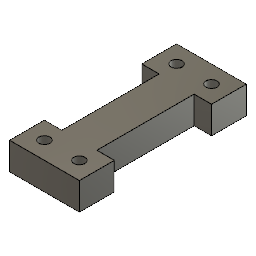
spacer_for_lbt-131_2mm (Autodesk Fusion 360 design; units mm, degrees)
Autodesk Fusion 360 part; units mm, degrees
note: some values were not read from the file. Set by a fixed rule: which sketch regions a step uses.
sketch "スケッチ1" plane through (0, 0, 0) normal (0, 1, 0) x (1, 0, 0)
  line L0 (0, 0) -> (0, 4.8)
  line L1 (0, 4.8) -> (1.27, 4.8)
  circle A0 centre (1.27, 4.8) radius 0.4
  circle A1 centre (-1.27, 4.8) radius 0.4
  circle A2 centre (-1.27, -4.8) radius 0.4
  circle A3 centre (1.27, -4.8) radius 0.4
  line L2 (-2.54, 3.53) -> (0, 3.53)
  line L3 (0, 3.53) -> (0, 6.07)
  line L4 (0, 6.07) -> (-2.54, 6.07)
  line L5 (-2.54, 6.07) -> (-2.54, 3.53)
  line L6 (-2.54, 3.53) -> (0, 6.07) construction
  line L7 (0, 3.53) -> (-2.54, 6.07) construction
  line L8 (2.54, 3.53) -> (0, 3.53)
  line L9 (2.54, 6.07) -> (2.54, 3.53)
  line L10 (0, 6.07) -> (2.54, 6.07)
  line L11 (0, 0) -> (1.27, 0)
  line L12 (-2.54, -3.53) -> (0, -3.53)
  line L13 (-2.54, -6.07) -> (-2.54, -3.53)
  line L14 (0, -6.07) -> (-2.54, -6.07)
  line L15 (0, -6.07) -> (2.54, -6.07)
  line L16 (2.54, -6.07) -> (2.54, -3.53)
  line L17 (2.54, -3.53) -> (0, -3.53)
  line L18 (1.27, 0) -> (1.27, 3.53)
  line L19 (-1.27, 0) -> (-1.27, 3.53)
  line L20 (1.27, 0) -> (1.27, -3.53)
  line L21 (-1.27, 0) -> (-1.27, -3.53)
  point P0 (-1.27, 4.8)
  dimension "d1" = 4.8
  dimension "d2" = 1.27
  dimension "d3" = 0.8
  dimension "d4" = 2.54
  dimension "d5" = 2.54
  dimension "d6" = 1.27
  constraint coincident L0.start L11.start
  constraint vertical L0
  constraint perpendicular L0 L1
  constraint coincident L1.end A0.centre
  constraint symmetric L0 A0 A1
  constraint perpendicular L2 L3
  constraint parallel L2 L4
  constraint parallel L3 L5
  constraint horizontal L2
  constraint coincident L6 P0
  constraint coincident L7 P0
  constraint coincident P0 A1.centre
  constraint symmetric L0 L2.start L8.start
  constraint symmetric L0 L2.end L3.start
  constraint symmetric L0 L3.end L4.start
  constraint symmetric L0 L4.end L9.start
  constraint perpendicular L0 L11
  constraint symmetric L2.start L11 L12.start
  constraint symmetric L2.end L11 L12.end
  constraint symmetric L3.end L11 L14.start
  constraint symmetric L4.end L11 L13.start
  constraint symmetric L8.start L11 L16.end
  constraint symmetric L9.start L11 L15.end
  constraint midpoint L8 L18.end
  constraint symmetric L0 L11.end L19.start
  constraint symmetric L0 L18.end L19.end
  constraint symmetric L18.start L11 L20.start
  constraint symmetric L11 L18.end L20.end
  constraint symmetric L11 L19.start L21.start
  constraint symmetric L11 L19.end L21.end
  measures "d1" distance of L0.start L0.end
  measures "d2" distance of L0.end L1.end
  measures "d3" diameter of A0
  measures "d4" distance of L2.end L3.end
  measures "d5" distance of L3.end L4.end
  measures "d6" distance of L0.start L11.end
extrude "押し出し1" add sketch "スケッチ1" along normal blind 2
